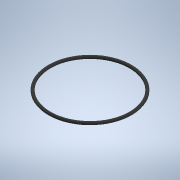
# Autodesk Inventor part: 2-240
Saved by Autodesk Inventor 2021 (Build 250183000, 183)
## iProperties
Created: 2021-10-18
Part Number: 2-240
Material: Rubber
Document SubType Name: Modeling
Designer: Alex Clay
Density: 0.93 g/cm^3
Appearance: Rubber - Black
Project: ODYSSEY
Mass: 2.81385 g
Surface Area: 34.2791 cm^2
Volume: 3.02565 cm^3
Author: Alex Clay
Comments: PARKER SIZE 2-240
Autodesk Inventor part; units mm, degrees
ref_plane "YZ Plane" through (0, 0, 0) normal (1, 0, 0) x (0, 1, 0)
ref_plane "XZ Plane" through (0, 0, 0) normal (0, 1, 0) x (-1, 0, 0)
ref_plane "XY Plane" through (0, 0, 0) normal (0, 0, 1) x (1, 0, 0)
sketch "Sketch1" plane through (0, 0, 0) normal (0, 0, 1) x (1, 0, 0)
  circle A0 centre (49.1871, 0) radius 1.7653
  line L0 (47.4218, 12.3168) -> (47.4218, -7.3576) construction
  line L1 (-10.1905, 0) -> (61.1429, 0) projected
  line L2 (0, -11.2924) -> (0, 16.2516) projected
  point P0 (0, 0)
  dimension "d0" = 47.4218
  dimension "d1" = 3.5306
  constraints: 2 end point, 1 centre point, 1 point on line, 1 tangent, 1 vertical
  measures "d0" distance from line of L0 point (0, 0)
  measures "d1" diameter of A0
revolve "Revolution1" add sketch "Sketch1" angle 360 about axis through (0, -10, 0) along (0, 1, 0)
body "Solid1"
